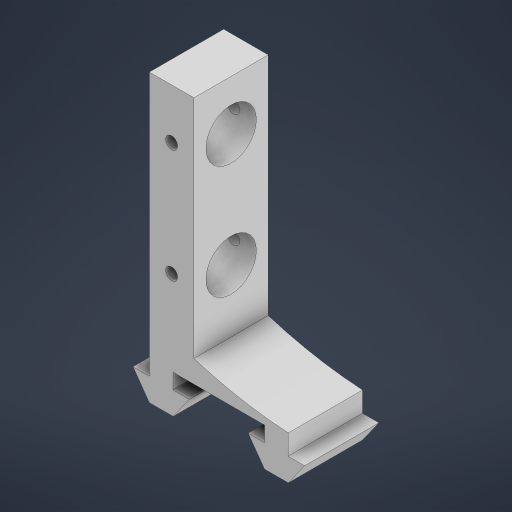
# Autodesk Inventor part: Part1
Saved by Autodesk Inventor 2023 (Build 270158000, 158)
## iProperties
Created: 2022-12-14
Part Number: Part1
Material: Generic
Document SubType Name: Modeling
Designer: CB110-09
Density: 1 g/cm^3
Appearance: Default
Author: CB110-09
Autodesk Inventor part; units mm, degrees
ref_plane "YZ Plane" through (0, 0, 0) normal (1, 0, 0) x (0, 1, 0)
ref_plane "XZ Plane" through (0, 0, 0) normal (0, 1, 0) x (-1, 0, 0)
ref_plane "XY Plane" through (0, 0, 0) normal (0, 0, 1) x (1, 0, 0)
sketch "Sketch1" plane through (0, 0, 0) normal (0, 0, 1) x (1, 0, 0)
  line L0 (4, 3.875) -> (-4, 3.875)
  line L1 (-4, 3.875) -> (-4, -3.875)
  line L2 (-4, -3.875) -> (4, -3.875)
  line L3 (4, -3.875) -> (4, 3.875)
  line L4 (4, 3.875) -> (-4, -3.875) construction
  line L5 (-4, 3.875) -> (4, -3.875) construction
  line L6 (4, 3.875) -> (9.5, 3.875)
  line L7 (-4, 3.875) -> (-9.5, 3.875)
  line L8 (4, -3.875) -> (9.5, 3.875)
  line L9 (-4, -3.875) -> (-9.5, 3.875)
  point P0 (0, 0)
  point P1 (0, 3.875)
  dimension "d0" = 8
  dimension "d1" = 7.75
  dimension "d2" = 9.5
  dimension "d3" = 9.5
  constraints: 20 end point, 3 horizontal, 3 midpoint, 2 parallel, 1 perpendicular
  measures "d0" distance of L2.end L1.end
  measures "d1" distance of L1.end L0.end
  measures "d2" distance of L6.end point (0, 3.875)
  measures "d3" distance of point (0, 3.875) L7.end
extrude "Extrusion1" add sketch "Sketch1" along normal blind 25
sketch "Sketch2" plane through (-9.5, 3.875, 0) normal (0, 1, 0) x (1, 0, 0)
  line L0 (0, 0) -> (5.5, 0) projected
  line L1 (5.5, -25) -> (13.5, -25) projected
  line L2 (5.5, 0) -> (5.5, -25)
  line L3 (5.5, -25) -> (13.5, -25)
  line L4 (13.5, 0) -> (19, 0) projected
  line L5 (13.5, -25) -> (13.5, 0)
  line L6 (5.5, 0) -> (13.5, 0) projected
  line L7 (13.5, 0) -> (5.5, 0)
  point P0 (9.5, 0)
  dimension "d6" = 8
  constraints: 8 end point, 2 collinear, 1 perpendicular, 1 vertical
  measures "d6" distance of L0.end L4.start
extrude "Extrusion2" add sketch "Sketch2" along normal blind 5
sketch "Sketch3" plane through (0, 0, 25) normal (0, 0, 1) x (1, 0, 0)
  line L0 (0, 0) -> (14.2258, 0)
  line L1 (-4, -3.875) -> (4, -3.875) projected
  line L2 (4, -3.875) -> (9.5, 3.875) projected
  line L3 (4, -3.875) -> (9.5, 3.875)
  line L4 (9.5, 3.875) -> (4, 3.875)
  line L5 (4, 3.875) -> (4, 8.875) projected
  line L6 (4, 3.875) -> (4, 8.875)
  line L7 (-4, 3.875) -> (-4, 8.875) projected
  line L8 (4, 8.875) -> (-4, 8.875)
  line L9 (-4, 8.875) -> (-4, 3.875)
  line L10 (-4, 3.875) -> (-9.5, 3.875) projected
  line L11 (-4, 3.875) -> (-9.5, 3.875)
  line L12 (-9.5, 3.875) -> (-4, -3.875)
  line L13 (42.75, -3.875) -> (48.25, 3.875)
  line L14 (48.25, 3.875) -> (42.75, 3.875)
  line L15 (42.75, 3.875) -> (42.75, 8.875)
  line L16 (42.75, 8.875) -> (34.75, 8.875)
  line L17 (34.75, 8.875) -> (34.75, 3.875)
  line L18 (34.75, 3.875) -> (29.25, 3.875)
  line L19 (29.25, 3.875) -> (34.75, -3.875)
  line L20 (34.75, -3.875) -> (42.75, -3.875)
  line L21 (34.75, 8.875) -> (42.75, 8.875)
  line L22 (42.75, 8.875) -> (42.75, 8.975)
  line L23 (42.75, 8.975) -> (34.75, 8.975)
  line L24 (34.75, 8.975) -> (34.75, 8.875)
  line L25 (4, 8.875) -> (-4, 8.875)
  line L26 (-4, 8.875) -> (-4, 8.975)
  line L27 (-4, 8.975) -> (4, 8.975)
  line L28 (4, 8.975) -> (4, 8.875)
  line L29 (-4, 8.975) -> (42.75, 8.975)
  line L30 (42.75, 8.975) -> (42.75, 10.675)
  line L31 (42.75, 10.675) -> (-4, 10.675)
  line L32 (-4, 10.675) -> (-4, 8.975)
  point P0 (6.75, 0)
  point P1 (38.75, 0)
  point P2 (52.9758, 0)
  point P3 (45.5, 0)
  dimension "d9" = 6.75
  dimension "d12" = 38.75
  dimension "d19" = 1.7
  dimension "d22" = 0.1
  constraints: 56 end point, 9 equal length, 7 horizontal, 5 perpendicular, 1 midpoint, 1 point on line, 18 other
  measures "d9" distance of point (6.75, 0) L0.start
  measures "d12" distance of L0.start point (38.75, 0)
  measures "d19" distance of L22.end L30.end
  measures "d22" distance of L22.end L21.end
extrude "Extrusion3" add sketch "Sketch3" against normal blind 25 contours L26 L27 L28 L8 | L23 L22 L16 L24 | L16 L15 L14 L13 L20 L19 L18 L17
extrude "Extrusion4" add sketch "Sketch3" against normal blind 25 contours L32 L31 L30 L23 L29 L27
sketch "Sketch4" plane through (0, 0, 25) normal (0, 0, 1) x (1, 0, 0)
  line L0 (42.75, 10.675) -> (-4, 10.675) projected
  line L1 (-4, 10.675) -> (42.75, 10.675)
  line L2 (42.75, 10.675) -> (42.75, 92.475)
  line L3 (42.75, 92.475) -> (-4, 92.475)
  line L4 (-4, 92.475) -> (-4, 10.675)
  line L5 (-4, 10.675) -> (11, 10.675)
  line L6 (11, 10.675) -> (11, 92.475)
  line L7 (11, 92.475) -> (-4, 92.475)
  line L8 (-4, 92.475) -> (-4, 10.675)
  line L9 (78.9241, 46.475) -> (-27.5343, 46.475)
  line L10 (-27.5343, 46.475) -> (-27.5343, 66.675)
  line L11 (-27.5343, 66.675) -> (78.9241, 66.675)
  line L12 (78.9241, 66.675) -> (78.9241, 46.475)
  line L13 (4, 8.975) -> (34.75, 8.975) projected
  line L14 (-36.8215, 45.475) -> (107.9586, 45.475)
  line L15 (107.9586, 45.475) -> (107.9586, 29.475)
  line L16 (107.9586, 29.475) -> (-36.8215, 29.475)
  line L17 (-36.8215, 29.475) -> (-36.8215, 45.475)
  line L18 (-39.8107, 67.675) -> (114.95, 67.675)
  line L19 (114.95, 67.675) -> (114.95, 83.675)
  line L20 (114.95, 83.675) -> (-39.8107, 83.675)
  line L21 (-39.8107, 83.675) -> (-39.8107, 67.675)
  point P0 (0, 0)
  dimension "d23" = 81.8
  dimension "d24" = 15
  dimension "d25" = 37.5
  dimension "d26" = 20.2
  dimension "d27" = 16
  dimension "d28" = 18.8
  dimension "d29" = 16
  dimension "d30" = 1
  dimension "d31" = 1
  dimension "d36" = 8.8
  dimension "d37" = 47
  constraints: 40 end point, 10 parallel, 5 horizontal, 5 perpendicular, 2 point on line
  measures "d23" distance of L1.end L2.end
  measures "d24" distance of L7.end L6.end
  measures "d25" distance between parallel lines of L9 L13
  measures "d26" distance between parallel lines of L11 L9
  measures "d27" distance of L14.end L15.end
  measures "d28" distance between parallel lines of L16 L0
  measures "d29" distance of L18.end L19.end
  measures "d30" distance between parallel lines of L9 L14
  measures "d31" distance between parallel lines of L18 L11
  measures "d36" distance between parallel lines of L20 L3
  measures "d37" distance between parallel lines of L14 L3
extrude "Extrusion5" add sketch "Sketch4" against normal blind 25 contours L0 L4 L16 L6 | L16 L4 L14 L6 | L14 L4 L9 L6 | L9 L4 L11 L6 | L11 L4 L18 L6 | L18 L4 L20 L6 | L20 L4 L3 L6
sketch "Sketch5" plane through (0, 0, 25) normal (0, 0, 1) x (1, 0, 0)
  line L0 (11, 92.475) -> (11, 10.675) projected
  line L1 (42.75, 10.675) -> (42.75, 3.875) projected
  arc A0 (11, 16.49) -> (42.75, 10.675) centre (50.7681, 144.0402) ccw
  line L2 (11, 16.49) -> (11, 10.675)
  line L3 (11, 10.675) -> (42.75, 10.675) projected
  line L4 (42.75, 10.675) -> (11, 10.675)
  line L5 (34.75, 8.975) -> (4, 8.975) projected
  point P0 (0, 0)
  constraints: 4 end point, 2 point on circle, 1 centre point, 1 parallel, 1 point on line, 1 vertical
extrude "Extrusion6" add sketch "Sketch5" against normal blind 25
sketch "Sketch6" plane through (-4, 3.875, 0) normal (-1, 0, 0) x (0, 0, 1)
  line L0 (25, 88.6) -> (0, 88.6) projected
  line L1 (25, 0) -> (25, 88.6) projected
  circle A0 centre (12.5, 71.8) radius 8.5
  circle A1 centre (12.5, 33.6) radius 8.5
  point P0 (0, -3.875)
  dimension "d38" = 16.8
  dimension "d39" = 12.5
  dimension "d40" = 17
  dimension "d41" = 55
  dimension "d42" = 17
  constraints: 2 centre point, 2 coincident
  measures "d38" distance from line of L0 point (12.5, 71.8)
  measures "d39" distance from line of L1 point (12.5, 71.8)
  measures "d40" diameter of A0
  measures "d41" distance from line of L0 point (12.5, 33.6)
  measures "d42" diameter of A1
extrude "Extrusion7" cut sketch "Sketch6" against normal blind 25
sketch "Sketch7" plane through (0, 0, 25) normal (0, 0, 1) x (1, 0, 0)
  line L0 (11, 16.49) -> (11, 92.475) projected
  line L1 (11, 92.475) -> (-4, 92.475) projected
  point P0 (0, 0)
  point P1 (3.5, 75.675)
  point P2 (3.5, 92.475)
  point P3 (3.5, 37.475)
  dimension "d45" = 7.5
  dimension "d46" = 16.8
  dimension "d47" = 55
  constraints: 1 midpoint
  measures "d45" distance from line of L0 point (3.5, 75.675)
  measures "d46" distance of point (3.5, 92.475) point (3.5, 75.675)
  measures "d47" distance from line of L1 point (3.5, 37.475)
hole "Hole1" at (3.5, 37.475, 25) at (3.5, 75.675, 25) direction (0, 0, -1) diameter 4 end through all
body "Solid1"
